Autodesk Inventor part; units mm, degrees
(part 2 of 2)
sketch "Sketch23" plane through (4.25, -2.86, 4.88) normal (0, 0, 1) x (1, 0, 0)
  line L0 (2, -1.15) -> (0, -1.15) projected
  line L1 (1.5, -1.15) -> (0.5, -1.15)
  line L2 (0.5, -1.15) -> (0.5, -0.65)
  line L3 (0.5, -0.65) -> (1.5, -0.65)
  line L4 (1.5, -0.65) -> (1.5, -1.15)
  line L5 (-9.45, -1.15) -> (-8.5, -1.15) projected
  line L6 (-9, -1.15) -> (-10, -1.15)
  line L7 (-10, -1.15) -> (-10, -0.65)
  line L8 (-10, -0.65) -> (-9, -0.65)
  line L9 (-9, -0.65) -> (-9, -1.15)
  line L10 (2, 0) -> (2, -1.15) projected
  line L11 (0, 0) -> (0, -1.15) projected
  line L12 (-10.5, 0) -> (-10.5, -1.15) projected
  line L13 (-8.5, 0) -> (-8.5, -1.15) projected
  point P0 (-4.25, 2.86)
  point P1 (0.5, -1.15)
  dimension "d337" = 1
  dimension "d338" = 0.5
  dimension "d339" = 1
  dimension "d340" = 0.5
  dimension "d341" = 0.5
  dimension "d342" = 0.5
  dimension "d343" = 0.5
  dimension "d344" = 0.5
  constraints: 16 end point, 4 parallel, 2 horizontal, 2 perpendicular, 2 point on line
  measures "d337" distance of L2.end L3.end
  measures "d338" distance of L1.end L2.end
  measures "d339" distance of L7.end L8.end
  measures "d340" distance of L6.end L7.end
  measures "d341" distance between parallel lines of L10 L4
  measures "d342" distance between parallel lines of L11 L2
  measures "d343" distance between parallel lines of L12 L7
  measures "d344" distance between parallel lines of L13 L9
extrude "Extrusion22" cut sketch "Sketch23" against normal blind 8
sketch "Sketch24" plane through (6.25, 0.32, -2.62) normal (1, 0, 0) x (0, 0, -1)
  line L0 (0.5, -3.83) -> (0.2, -3.83) projected
  line L1 (-7.5, -3.83) -> (0.5, -3.83) projected
  line L2 (-7.5, -3.83) -> (0.2, -3.83) projected
  line L3 (-7.5, -3.18) -> (-7.5, -4.33) projected
  line L4 (-7.5, -3.505) -> (-5.06, -3.18)
  line L5 (-7.5, -3.18) -> (-2.62, -3.18) projected
  line L6 (-5.06, -3.18) -> (-7.5, -3.18)
  line L7 (-7.5, -3.18) -> (-7.5, -3.505)
  dimension "d347" = 0.325
  dimension "d348" = 0.325
  constraints: 6 end point, 1 collinear, 1 midpoint, 1 perpendicular, 1 point on line
  measures "d347" distance from line of L4.start L1
  measures "d348" distance from line of L5 L4.start
extrude "Extrusion23" cut sketch "Sketch24" against normal up to surface (12.5 mm away)
chamfer "Chamfer1" distance 0.28 angle 45 20 edges at (4, 0, 8) (2, 0, 8) (0, 0, 8) (-2, 0, 8) (-4, 0, 8) (1.395, 0, 8.775) (2.605, 0, 8.775) (-0.605, 0, 8.775) (0.605, 0, 8.775) (-1.395, 0, 8.775) (-2.605, 0, 8.775) (-3.395, 0, 8.775) (-4.605, 0, 8.775) (3.395, 0, 8.775) (4.605, 0, 8.775) (2, 0, 9.55) (0, 0, 9.55) (-2, 0, 9.55) (-4, 0, 9.55) (4, 0, 9.55)
sketch "Sketch25" plane through (5.55, 0, 9.284) normal (1, 0, 0) x (0, 0, -1)
  line L0 (-0.866, 0) -> (-0.866, 1.84) projected
  line L1 (-0.866, 0) -> (-0.866, 0.38)
  line L2 (-0.866, 0.38) -> (-0.2078, 0)
  line L3 (-0.2078, 0) -> (-0.866, 0)
  line L4 (-0.866, 1.84) -> (0, 1.84) projected
  line L5 (-0.866, 1.84) -> (-0.866, 1.34)
  line L6 (0, 1.84) -> (9.284, 1.84) projected
  line L7 (-0.866, 1.34) -> (0, 1.84)
  line L8 (0, 1.84) -> (-0.866, 1.84)
  line L9 (0, 0) -> (9.284, 0) projected
  point P0 (-0.866, 1.34)
  dimension "d355" = 0.38
  dimension "d356" = 60
  dimension "d357" = 0.5
  dimension "d358" = 60
  constraints: 12 end point, 2 collinear, 2 point on line
  measures "d355" distance of L0.start L1.end
  measures "d356" angle of L1 L2
  measures "d357" distance of L0.end L5.end
  measures "d358" angle of L7 L5
extrude "Extrusion24" cut sketch "Sketch25" against normal up to surface (11.1 mm away)
fillet "Fillet1" radius 0.1 4 edges at (-6.4, 0.32, -2.62) (-6.4, -0.68, -2.62) (6.4, 0.32, -2.62) (6.4, -0.68, -2.62)
fillet "Fillet1" radius 0.5 2 edges at (5.55, 1.84, 4.642) (-5.55, 1.84, 4.642)
fillet "Fillet1" radius 0.2 2 edges at (-6.25, 2.56, -2.31) (6.25, 2.56, -2.31)
equation "\"d9\" = d8"
equation "\"d19\" = d17"
equation "\"d20\" = d18"
equation "\"d35\" = d34"
equation "\"d96\" = d97"
equation "\"d99\" = d95"
equation "\"d100\" = d95"
equation "\"d101\" = d95"
equation "\"d102\" = d95"
equation "\"d103\" = d104"
equation "\"d105\" = d106"
equation "\"d107\" = d108"
equation "\"d109\" = d110"
equation "\"d114\" = d113"
equation "\"d32\" = d33"
equation "\"d33\" = 0.8"
body "Solid1"
